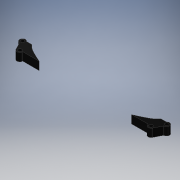
# Autodesk Inventor part: LightGate
Saved by Autodesk Inventor 2017 (Build 210142000, 142)
## iProperties
Created: 2019-03-18
Part Number: LightGate
Material: Generic
Document SubType Name: Modeling
Designer: cresswnd
Density: 1 g/cm^3
Appearance: Glossy - Black
Author: cresswnd
Autodesk Inventor part; units mm, degrees
ref_plane "YZ Plane" through (0, 0, 0) normal (1, 0, 0) x (0, 1, 0)
ref_plane "XZ Plane" through (0, 0, 0) normal (0, 1, 0) x (-1, 0, 0)
ref_plane "XY Plane" through (0, 0, 0) normal (0, 0, 1) x (1, 0, 0)
sketch "Sketch1" plane through (0, 0, 0) normal (0, 0, 1) x (1, 0, 0)
  circle A0 centre (-17.5, 50.3933) radius 1.5 projected
  circle A1 centre (17.5019, 50.3933) radius 1.5 projected
  circle A2 centre (-92.4889, 4.8422) radius 1.5 projected
  circle A3 centre (92.5009, 4.8422) radius 1.5 projected
  circle A4 centre (12.5035, -31.0904) radius 1.5 projected
  circle A5 centre (-22.4965, -50.3404) radius 1.5 projected
  circle A6 centre (22.5035, -50.3404) radius 1.5 projected
  circle A7 centre (-12.4965, -31.0904) radius 1.5 projected
  circle A8 centre (-13.0811, 17.9237) radius 1.5 projected
  circle A9 centre (13.0818, -8.2392) radius 1.5 projected
  circle A10 centre (-13.0811, -8.2392) radius 1.5 projected
  circle A11 centre (13.0818, 17.9237) radius 1.5 projected
  arc A12 (40.7538, -8.8872) -> (25.4622, 39.5007) centre (0.0036, 4.845) ccw projected
  arc A13 (33.5156, -11.6206) -> (40.7538, -8.8872) centre (36.0156, -7.2905) ccw projected
  line L0 (33.5156, -11.6206) -> (19.6226, -3.5994) projected
  arc A14 (17.2069, 1.645) -> (19.6226, -3.5994) centre (22.1226, 0.7307) ccw projected
  arc A15 (17.2069, 1.645) -> (17.502, 4.845) centre (0.0036, 4.845) ccw projected
  line L1 (17.502, 4.845) -> (17.502, 35.4711) projected
  arc A16 (25.4622, 39.5007) -> (17.502, 35.4711) centre (22.502, 35.4711) ccw projected
  line L2 (-19.6207, -3.5985) -> (-33.5095, -11.6173) projected
  arc A17 (-40.7478, -8.8835) -> (-33.5095, -11.6173) centre (-36.0095, -7.2872) ccw projected
  arc A18 (-25.4608, 39.4964) -> (-40.7478, -8.8835) centre (0.0036, 4.845) ccw projected
  arc A19 (-17.4999, 35.4673) -> (-25.4608, 39.4964) centre (-22.4999, 35.4673) ccw projected
  line L3 (-17.4999, 35.4673) -> (-17.4999, 4.845) projected
  arc A20 (-17.4999, 4.845) -> (-17.205, 1.6455) centre (0.0036, 4.845) ccw projected
  arc A21 (-19.6207, -3.5985) -> (-17.205, 1.6455) centre (-22.1208, 0.7316) ccw projected
  arc A22 (73.7428, 35.443) -> (75.5899, 34.722) centre (75.6959, 37.7202) ccw projected
  arc A23 (77.3954, 33.4159) -> (75.5899, 34.722) centre (75.5192, 32.7233) ccw projected
  arc A24 (73.6411, -32.348) -> (77.3954, 33.4159) centre (0.0036, 4.845) ccw projected
  arc A25 (70.8559, -33.1784) -> (73.6411, -32.348) centre (71.8559, -31.4463) ccw projected
  line L4 (70.8559, -33.1784) -> (61.2941, -27.6579) projected
  arc A26 (60.501, -25.04) -> (61.2941, -27.6579) centre (62.2941, -25.9258) ccw projected
  arc A27 (60.501, -25.04) -> (63.0565, 28.8737) centre (0.0036, 4.845) ccw projected
  arc A28 (63.9254, 31.318) -> (63.0565, 28.8737) centre (64.9254, 29.5859) ccw projected
  line L5 (63.9254, 31.318) -> (71.4407, 35.657) projected
  arc A29 (73.7428, 35.443) -> (71.4407, 35.657) centre (72.4407, 33.9249) ccw projected
  arc A30 (-77.3818, 33.4198) -> (-73.6297, -32.3457) centre (0.0036, 4.845) ccw projected
  arc A31 (-75.5839, 34.7254) -> (-77.3818, 33.4198) centre (-75.5056, 32.727) ccw projected
  arc A32 (-75.5839, 34.7254) -> (-73.7475, 35.4465) centre (-75.7012, 37.7231) ccw projected
  arc A33 (-71.445, 35.6608) -> (-73.7475, 35.4465) centre (-72.445, 33.9288) ccw projected
  line L6 (-71.445, 35.6608) -> (-63.9219, 31.3173) projected
  arc A34 (-63.053, 28.8731) -> (-63.9219, 31.3173) centre (-64.9219, 29.5853) ccw projected
  arc A35 (-63.053, 28.8731) -> (-60.4965, -25.0417) centre (0.0036, 4.845) ccw projected
  arc A36 (-61.2897, -27.6596) -> (-60.4965, -25.0417) centre (-62.2897, -25.9275) ccw projected
  line L7 (-61.2897, -27.6596) -> (-70.8445, -33.1761) projected
  arc A37 (-73.6297, -32.3457) -> (-70.8445, -33.1761) centre (-71.8445, -31.444) ccw projected
  arc A38 (84.1399, 28.8587) -> (62.8691, 65.7009) centre (0.0003, 4.8422) ccw projected
  arc A39 (63.5246, 70.3855) -> (62.8691, 65.7009) centre (65.0246, 67.7874) ccw projected
  line L8 (63.5246, 70.3855) -> (69.3166, 73.7296) projected
  arc A40 (73.0068, 73.1816) -> (69.3166, 73.7296) centre (70.8166, 71.1315) ccw projected
  arc A41 (95.687, 33.8976) -> (73.0068, 73.1816) centre (0.0036, 4.845) ccw projected
  arc A42 (94.3164, 30.4279) -> (95.687, 33.8976) centre (92.8164, 33.026) ccw projected
  line L9 (94.3164, 30.4279) -> (88.5247, 27.0841) projected
  arc A43 (84.1399, 28.8587) -> (88.5247, 27.0841) centre (87.0246, 29.6822) ccw projected
  line L10 (-88.5239, 27.0841) -> (-94.3153, 30.4277) projected
  arc A44 (-95.6859, 33.8974) -> (-94.3153, 30.4277) centre (-92.8153, 33.0258) ccw projected
  arc A45 (-73.0058, 73.1815) -> (-95.6859, 33.8974) centre (0.0007, 4.8432) ccw projected
  arc A46 (-69.3155, 73.7294) -> (-73.0058, 73.1815) centre (-70.8156, 71.1313) ccw projected
  line L11 (-69.3155, 73.7294) -> (-63.5239, 70.3855) projected
  arc A47 (-62.8684, 65.7008) -> (-63.5239, 70.3855) centre (-65.0239, 67.7874) ccw projected
  arc A48 (-62.8684, 65.7008) -> (-84.1392, 28.8588) centre (0.0004, 4.8422) ccw projected
  arc A49 (-88.5239, 27.0841) -> (-84.1392, 28.8588) centre (-87.0239, 29.6822) ccw projected
  arc A50 (-22.6799, -92.551) -> (22.679, -92.5515) centre (0.0006, 4.8432) ccw projected
  arc A51 (-24.9995, -89.6292) -> (-22.6799, -92.551) centre (-21.9995, -89.6292) ccw projected
  line L12 (-24.9995, -89.6292) -> (-24.9996, -82.9431) projected
  arc A52 (-21.2703, -80.033) -> (-24.9996, -82.9431) centre (-21.9996, -82.943) ccw projected
  arc A53 (-21.2703, -80.033) -> (21.2694, -80.0334) centre (0.0003, 4.8422) ccw projected
  arc A54 (24.9986, -82.9434) -> (21.2694, -80.0334) centre (21.9986, -82.9434) ccw projected
  line L13 (24.9986, -82.9434) -> (24.9986, -89.6296) projected
  arc A55 (22.679, -92.5515) -> (24.9986, -89.6296) centre (21.9986, -89.6296) ccw projected
  circle A56 centre (0.0003, 4.8422) radius 12.5 projected
  circle A57 centre (-75.7012, 37.7231) radius 1.45 projected
  circle A58 centre (-66.3185, 53.9572) radius 1.45 projected
  circle A59 centre (66.3269, 53.9611) radius 1.45 projected
  circle A60 centre (75.6959, 37.7202) radius 1.45 projected
  circle A61 centre (9.3764, -77.1476) radius 1.45 projected
  circle A62 centre (-9.3746, -77.1579) radius 1.45 projected
  arc A63 (-60.75, 88.6314) -> (-62.3386, 89.3348) centre (-61.7449, 88.5301) ccw projected
  arc A64 (-62.3386, 89.3348) -> (62.3383, 89.3352) centre (0.0001, 4.8424) ccw projected
  arc A65 (62.3383, 89.3352) -> (60.7498, 88.6319) centre (61.7446, 88.5305) ccw projected
  arc A66 (53.8357, 75.1858) -> (55.8157, 77.1858) centre (40.1318, 90.7331) ccw
  arc A67 (-55.6054, 76.9436) -> (-53.7905, 75.1436) centre (-40.131, 90.7312) ccw
  circle A68 centre (9.5003, 29.8384) radius 1.5 projected
  circle A69 centre (15.0012, -19.6648) radius 1.5 projected
  circle A70 centre (9.5003, 42.3384) radius 1.5 projected
  circle A71 centre (15.0012, 4.8446) radius 1.5 projected
  circle A72 centre (-15.0005, 4.8446) radius 1.5 projected
  circle A73 centre (-9.4997, 42.3384) radius 1.5 projected
  circle A74 centre (-15.0005, -19.6648) radius 1.5 projected
  circle A75 centre (-9.4997, 29.8384) radius 1.5 projected
  circle A76 centre (56.5857, 67.6399) radius 1.5
  circle A77 centre (-56.5856, 67.6399) radius 1.5
  circle A78 centre (-62.1259, 75.5523) radius 1.5
  circle A79 centre (62.126, 75.5523) radius 1.5
  circle A80 centre (-18.1771, -30.5421) radius 1.5 projected
  circle A81 centre (-86.5108, -45.1051) radius 1.5 projected
  circle A82 centre (86.5116, -45.1051) radius 1.5 projected
  circle A83 centre (18.1778, -30.5421) radius 1.5 projected
  circle A84 centre (58.291, 73.7158) radius 0.51 projected
  circle A85 centre (58.2919, 71.1758) radius 0.51 projected
  circle A86 centre (-58.289, 73.6736) radius 0.51 projected
  circle A87 centre (-58.288, 71.1336) radius 0.51 projected
  arc A88 (-60.0488, 76.9436) -> (-62.1259, 73.0523) centre (-62.1259, 75.5523) ccw
  arc A89 (-58.8163, 66.5113) -> (-55.1184, 69.6641) centre (-56.5856, 67.6399) ccw
  line L14 (-62.1259, 73.0523) -> (-58.8163, 66.5113)
  line L15 (-60.0488, 76.9436) -> (-55.6054, 76.9436)
  line L16 (-55.1184, 69.6641) -> (-58.0529, 69.6641)
  line L17 (-55.1184, 69.6641) -> (-59.8377, 69.6641)
  line L18 (-59.8377, 75.1436) -> (-59.8377, 69.6641)
  line L19 (-59.8377, 75.1436) -> (-53.7905, 75.1436)
  line L20 (-55.1184, 69.6641) -> (-44.3518, 69.6641)
  line L21 (-39.7789, 67.6641) -> (-54.0857, 67.6641)
  arc A90 (54.0866, 67.7058) -> (58.8164, 66.5113) centre (56.5857, 67.6399) ccw
  arc A91 (62.126, 73.0523) -> (60.2334, 77.1858) centre (62.126, 75.5523) ccw
  line L22 (55.8157, 77.1858) -> (60.2334, 77.1858)
  line L23 (59.5645, 72.4463) -> (59.7645, 72.4463)
  line L24 (59.7645, 69.7058) -> (59.7645, 75.1858)
  line L25 (53.8357, 75.1858) -> (59.7645, 75.1858)
  line L26 (59.7645, 69.7058) -> (44.4365, 69.7058)
  line L27 (39.7895, 67.6704) -> (54.0866, 67.7058)
  line L28 (62.126, 73.0523) -> (58.8164, 66.5113)
  arc A92 (-44.3518, 69.6641) -> (-39.7789, 67.6641) centre (-0.0023, 164.8397) ccw
  arc A93 (39.7895, 67.6704) -> (44.4365, 69.7058) centre (-0.0023, 164.8397) ccw
  point P0 (0, 0)
  dimension "d2" = 5
  dimension "d5" = 5
  dimension "d12" = 5
  dimension "d13" = 5
  dimension "d16" = 0.2
  constraints: 30 end point, 17 point on circle, 12 centre point, 10 horizontal, 4 coincident, 2 tangent, 2 vertical
  measures "d2" diameter of A88
  measures "d5" diameter of A89
  measures "d12" diameter of A90
  measures "d13" diameter of A91
  measures "d16" distance of L23.start L23.end
extrude "Extrusion2" add sketch "Sketch1" along normal blind 5.5 contours A66 L22 A91 L28 A90 L27 A93 L26 L24 L25 | A67 L19 L18 L17 L16 A89 L14 A88 L15 | A89 L20 A92 L21
sketch "Sketch2" plane through (0, 0, 5.5) normal (0, 0, 1) x (1, 0, 0)
  arc A0 (-55.6064, 76.9436) -> (-50.0015, 72.5062) centre (-40.1324, 90.7302) ccw
  arc A1 (50.0011, 72.5081) -> (55.8157, 77.1858) centre (40.1304, 90.7307) ccw
  circle A2 centre (62.126, 75.5523) radius 1.5 projected
  circle A3 centre (56.5857, 67.6399) radius 1.5 projected
  line L0 (39.7895, 67.6704) -> (54.0866, 67.7058) projected
  arc A4 (54.0866, 67.7058) -> (58.8164, 66.5113) centre (56.5857, 67.6399) ccw projected
  line L1 (58.8164, 66.5113) -> (62.126, 73.0523) projected
  arc A5 (62.126, 73.0523) -> (60.2334, 77.1858) centre (62.126, 75.5523) ccw projected
  line L2 (60.2334, 77.1858) -> (55.8157, 77.1858)
  circle A6 centre (-62.1259, 75.5523) radius 1.5 projected
  circle A7 centre (-56.5856, 67.6399) radius 1.5 projected
  line L3 (-55.6054, 76.9436) -> (-60.0488, 76.9436) projected
  arc A8 (-60.0488, 76.9436) -> (-62.1259, 73.0523) centre (-62.1259, 75.5523) ccw projected
  line L4 (-62.1259, 73.0523) -> (-58.8163, 66.5113) projected
  arc A9 (-58.8163, 66.5113) -> (-54.0857, 67.6641) centre (-56.5856, 67.6399) ccw projected
  line L5 (-54.0857, 67.6641) -> (-39.7789, 67.6641) projected
  arc A10 (-50.0015, 72.5062) -> (-39.781, 67.6641) centre (-0.0004, 164.838) ccw
  arc A11 (39.7917, 67.6704) -> (50.0011, 72.5081) centre (-0.0004, 164.838) ccw
  point P0 (0, 0)
  point P1 (59.7645, 69.7058)
  constraints: 12 centre point, 8 point on circle, 3 point on line, 2 end point, 3 other
extrude "Extrusion4" add sketch "Sketch2" along normal blind 1.5
sketch "Sketch4" plane through (0, 0, 0) normal (1, 0, 0) x (0, 1, 0)
  line L0 (75.1436, 0) -> (75.1436, 5.5)
  line L1 (69.6641, 5.5) -> (75.1436, 5.5)
  line L2 (69.6641, 0) -> (69.6641, 5.5)
  line L3 (69.6641, 0) -> (69.6641, 5.5) projected
  arc A0 (75.0038, 2.75) -> (69.8038, 2.75) centre (72.4038, 2.75) ccw
  line L4 (69.8038, 2.75) -> (69.8038, 0)
  line L5 (75.0038, 2.75) -> (75.0038, 0)
  line L6 (69.6641, 0) -> (69.8038, 0)
  line L7 (75.0038, 0) -> (75.1436, 0)
  point P0 (0, 0)
  dimension "d25" = 5.2
  constraints: 14 end point, 4 perpendicular, 2 point on circle, 1 centre point, 1 tangent
  measures "d25" diameter of A0
extrude "Extrusion5" add sketch "Sketch4" along normal mid plane 120
sketch "Sketch5" plane through (0, 0, 7) normal (0, 0, 1) x (1, 0, 0)
  arc A0 (50.0011, 72.5081) -> (55.8157, 77.1858) centre (40.1304, 90.7307) ccw projected
  arc A1 (39.7917, 67.6704) -> (50.0011, 72.5081) centre (-0.0004, 164.838) ccw projected
  arc A2 (39.7895, 67.6704) -> (44.3471, 69.6641) centre (-0.0023, 164.8397) ccw projected
  line L0 (39.7895, 67.6704) -> (39.7917, 67.6704) projected
  arc A3 (39.7917, 67.6704) -> (50.0011, 72.5081) centre (-0.0004, 164.838) ccw projected
  arc A4 (50.0011, 72.5081) -> (53.7882, 75.1436) centre (40.1304, 90.7307) ccw projected
  line L1 (-53.7905, 75.1436) -> (53.7882, 75.1436) projected
  arc A5 (-55.6054, 76.9436) -> (-53.7905, 75.1436) centre (-40.131, 90.7312) ccw projected
  line L2 (-55.6054, 76.9436) -> (-55.6064, 76.9436) projected
  arc A6 (-55.6064, 76.9436) -> (-50.0015, 72.5062) centre (-40.1324, 90.7302) ccw projected
  arc A7 (-50.0015, 72.5062) -> (-39.781, 67.6641) centre (-0.0004, 164.838) ccw projected
  line L3 (-39.781, 67.6641) -> (-39.7789, 67.6641) projected
  arc A8 (-44.3518, 69.6641) -> (-39.7789, 67.6641) centre (-0.0023, 164.8397) ccw projected
  line L4 (-44.3518, 69.6641) -> (44.3471, 69.6641) projected
  point P0 (0, 0)
extrude "Extrusion6" cut sketch "Sketch5" against normal blind 20
body "Solid2"
